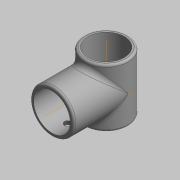
# Autodesk Inventor part: L10-6
Saved by Autodesk Inventor 2019.4 (Build 234330000, 330)
## iProperties
Created: 2020-04-23
Part Number: L10-6
Material: Generic
Document SubType Name: Modeling
Designer: Hannah
Density: 1 g/cm^3
Appearance: Default
Author: Hannah
Autodesk Inventor part; units mm, degrees
ref_plane "XY Plane" through (0, 0, 0) normal (0, 0, 1) x (1, 0, 0)
sketch "Sketch1" plane through (0, 0, 0) normal (0, 0, 1) x (1, 0, 0)
  circle A0 centre (0, 0) radius 17.5
  circle A1 centre (0, 0) radius 21
  dimension "d1" = 42
  dimension "d2" = 35
  constraints: 2 centre point, 2 coincident
  measures "d1" diameter of A1
  measures "d2" diameter of A0
extrude "Extrusion1" add sketch "Sketch1" along normal blind 52 contours A0 | A1
sketch "Sketch2" plane through (0, 0, 0) normal (0, 1, 0) x (-1, 0, 0)
  circle A0 centre (0, 0) radius 17.5
  circle A1 centre (0, 0) radius 21
  dimension "d5" = 35
  dimension "d6" = 42
  constraints: 2 centre point, 2 coincident
  measures "d5" diameter of A0
  measures "d6" diameter of A1
extrude "Extrusion2" add sketch "Sketch2" along normal mid plane 56 contours A0 | A1
extrude "Extrusion3" cut sketch "Sketch2" against normal up to surface (56 mm away) from surface at 28 contours A0
extrude "Extrusion4" cut sketch "Sketch1" along normal up to surface (52 mm away) contours A0
fillet "Fillet1" radius 5 2 edges at (0, 21, 21) (0, -21, 21)
hole "Hole1" at (0, 0, 0) direction (-1, 0, 0) diameter 6.647 end through all thread size "M8x1.25" class "6H" standard "ISO Metric profile"
ref_plane "Work Plane1" through (0, 0, 36.5) normal (0, 0, 1) x (1, 0, 0)
hole "Hole2" at (0, 0, 36.5) direction (0, -1, 0) diameter 6.647 end through all thread size "M8x1.25" class "6H" standard "ISO Metric profile"
fillet "Fillet2" radius 2 3 edges at (21, 28, 0) (-21, 0, 52) (21, -28, 0)
equation "\"d5\" = d2"
equation "\"d6\" = d1"
equation "\"d23\" = -0.5 * d3 + 0.25 * d1"
equation "\"d3\" = 52"
body "Solid1"
